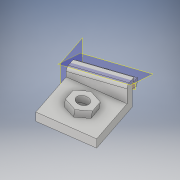
# Autodesk Inventor part: sem2_thumbmount2
Saved by Autodesk Inventor 2018 (Build 220112000, 112)
## iProperties
Created: 2018-01-19
Part Number: sem2_thumbmount2
Material: Generic
Document SubType Name: Modeling
Designer: rheal
Density: 1 g/cm^3
Appearance: Default
Author: rheal
Autodesk Inventor part; units mm, degrees
ref_plane "YZ Plane" through (0, 0, 0) normal (1, 0, 0) x (0, 1, 0)
ref_plane "XZ Plane" through (0, 0, 0) normal (0, 1, 0) x (-1, 0, 0)
ref_plane "XY Plane" through (0, 0, 0) normal (0, 0, 1) x (1, 0, 0)
ref_plane "Work Plane2" through (-15, 5, -15) normal (-0.9487, 0, 0.3162) x (0, -1, 0)
sketch "Sketch3" plane through (-15, 5, -15) normal (-0.9487, 0, 0.3162) x (0, -1, 0)
  line L0 (0, 37.9473) -> (0, 0) projected
  line L1 (0, 0) -> (-5, 0)
  line L2 (-5, 0) -> (-5, 3)
  line L3 (-3, 5) -> (0, 5)
  line L4 (0, 0) -> (0, 5)
  arc A0 (-3, 5) -> (-5, 3) centre (-3, 3) ccw
  line L5 (0, 0) -> (5.0254, 0) construction
  line L6 (5, 0) -> (0, 0) projected
  line L7 (0, 0) -> (-5, -1.8199)
  line L8 (0, 0) -> (5.3209, 0) construction
  line L9 (-5, -1.8199) -> (-5, 0)
  line L10 (0, 0) -> (-3.2889, -1.1971)
  line L11 (0, 0) -> (-2.8191, -1.0261)
  line L12 (0, 0) -> (1.5391, -4.2286)
  line L13 (1.5391, -4.2286) -> (-2.6895, -5.7677)
  line L14 (-2.6895, -5.7677) -> (-2.8191, -1.0261)
  point P0 (5, 18.9737)
  point P1 (-5, 5)
  dimension "d5" = 5
  dimension "d6" = 5
  dimension "d7" = 2
  dimension "d9" = 160
  dimension "d12" = 3.5
  dimension "d20" = 3
  dimension "d21" = 4.5
  constraints: 26 end point, 5 perpendicular, 5 point on line, 3 horizontal, 2 point on circle, 2 tangent, 1 centre point, 1 equal length
  measures "d5" distance of L0.end L1.end
  measures "d6" distance of L1.end point (-5, 5)
  measures "d7" radius of A0
  measures "d9" angle of L7 L8
  measures "d12" distance of L0.end L10.end
  measures "d20" distance of L0.end L11.end
  measures "d21" distance of L0.end L12.end
extrude "Extrusion2" add sketch "Sketch3" against normal blind 30
ref_plane "Work Plane4" through (-16.8239, 7.6895, -20.4717) normal (0.1082, -0.9397, 0.3245) x (0.9487, 0, -0.3162)
sketch "Sketch5" plane through (-16.8239, 7.6895, -20.4717) normal (0.1082, -0.9397, 0.3245) x (0.9487, 0, -0.3162)
  line L0 (30, 4.5) -> (30, 0) projected
  line L1 (30, 0) -> (30, -0.5)
  line L2 (30, -0.5) -> (15, -0.5)
  line L3 (15, -0.5) -> (15, 2)
  circle A0 centre (15, 2) radius 1.5
  point P0 (9.4868, 20.6193)
  dimension "d24" = 0.5
  dimension "d25" = 15
  dimension "d26" = 2.5
  dimension "d27" = 3
  constraints: 6 end point, 2 perpendicular, 1 centre point, 1 coincident, 1 vertical
  measures "d24" distance of L0.end L1.end
  measures "d25" distance of L1.end L2.end
  measures "d26" distance of L2.end L3.end
  measures "d27" diameter of A0
extrude "Extrusion4" cut sketch "Sketch5" along normal blind 10
sketch "Sketch7" plane through (-15, 5, -15) normal (-0.9487, 0, 0.3162) x (0, -1, 0)
  line L0 (0, 0) -> (6.5506, 2.3842)
  line L1 (0, 0) -> (6.971, 0) construction
  line L2 (6.5506, 2.3842) -> (6.5506, -3.325)
  line L3 (6.5506, -3.325) -> (0, 0)
  point P0 (5, 18.9737)
  dimension "d34" = 20
  constraints: 8 end point, 1 equal length, 1 horizontal, 1 vertical
  measures "d34" angle of L1 L0
extrude "Extrusion6" cut sketch "Sketch7" along normal blind 5 and the other way blind 40
fillet "Fillet2" radius 0.5 1 edges at (-2.5937, 7.6895, -25.2151)
sketch "Sketch8" plane through (-13.4189, 5, -10.2566) normal (0.3162, 0, 0.9487) x (0.9487, 0, -0.3162)
  line L0 (30, 0) -> (31.6228, 0) projected
  line L1 (30, 0) -> (36.1043, 0)
  line L2 (36.1043, 0) -> (36.1043, -10.0041)
  line L3 (36.1043, -10.0041) -> (30, -10.0041)
  line L4 (30, -10.0041) -> (30, 0)
  point P0 (9.4868, -5)
  constraints: 8 end point, 2 parallel, 1 horizontal, 1 perpendicular
extrude "Extrusion7" cut sketch "Sketch8" along normal mid plane 20
ref_plane "Work Plane7" through (-15, 5, -15) normal (0.3162, 0, 0.9487) x (0.9487, 0, -0.3162)
sketch "Sketch10" plane through (-15, 5, -15) normal (0.3162, 0, 0.9487) x (0.9487, 0, -0.3162)
  line L0 (0, 0) -> (30, 0) projected
  line L1 (0, 0) -> (30, 0)
  line L2 (30, 0) -> (30, -5)
  line L3 (30, -5) -> (0, -5)
  line L4 (0, -5) -> (0, 0)
  line L5 (30, -5) -> (30, -10)
  line L6 (30, -10) -> (0, -5)
  point P0 (9.4868, -5)
  dimension "d49" = 30
  dimension "d50" = 5
  dimension "d51" = 5
  constraints: 12 end point, 2 parallel, 1 horizontal, 1 perpendicular, 1 vertical
  measures "d49" distance of L2.end L3.end
  measures "d50" distance of L1.end L2.end
  measures "d51" distance of L2.end L5.end
extrude "Extrusion8" add sketch "Sketch10" along normal blind 5
sketch "Sketch11" plane through (15.0416, -5, -19.7434) normal (0.3162, 0, 0.9487) x (0.9487, 0, -0.3162)
  line L0 (-30, 10) -> (-30, 5) projected
  line L1 (-30, 5) -> (-30, 10)
  line L2 (-30, 10) -> (0, 5)
  line L3 (0, 0) -> (0, 10) projected
  line L4 (0, 0) -> (0, 5)
  line L5 (-30, 5) -> (0, 0) projected
  line L6 (0, 0) -> (-30, 5)
  point P0 (-20.5132, 5)
  dimension "d54" = 5
  constraints: 8 end point, 3 collinear, 1 midpoint
  measures "d54" distance of L0.end L0.start
extrude "Extrusion9" add sketch "Sketch11" along normal blind 30
sketch "Sketch13" plane through (-13.4189, 5, -10.2566) normal (0.156, 0.9864, -0.052) x (0.9358, -0.1644, -0.3119)
  line L0 (30.4138, -30) -> (0, -30) projected
  line L1 (15.2069, -30) -> (15.2069, -15)
  circle A0 centre (15.2069, -15) radius 6.75
  line L2 (21.9569, -18.8971) -> (15.2069, -22.7942)
  line L3 (15.2069, -22.7942) -> (8.4569, -18.8971)
  line L4 (8.4569, -18.8971) -> (8.4569, -11.1029)
  line L5 (8.4569, -11.1029) -> (15.2069, -7.2058)
  line L6 (15.2069, -7.2058) -> (21.9569, -11.1029)
  line L7 (21.9569, -11.1029) -> (21.9569, -18.8971)
  circle A1 centre (15.2069, -15) radius 3.5
  point P0 (10.1797, -13.9737)
  point P1 (21.9569, -15)
  dimension "d58" = 13.5
  dimension "d57" = 15
  dimension "d59" = 7
  constraints: 14 end point, 3 coincident, 2 midpoint, 1 centre point, 1 horizontal alignment, 1 vertical, 15 other
  measures "d57" distance of L1.start L1.end
  measures "d59" diameter of A1
extrude "Extrusion10" add sketch "Sketch13" along normal blind 4.25
body "Solid1"
